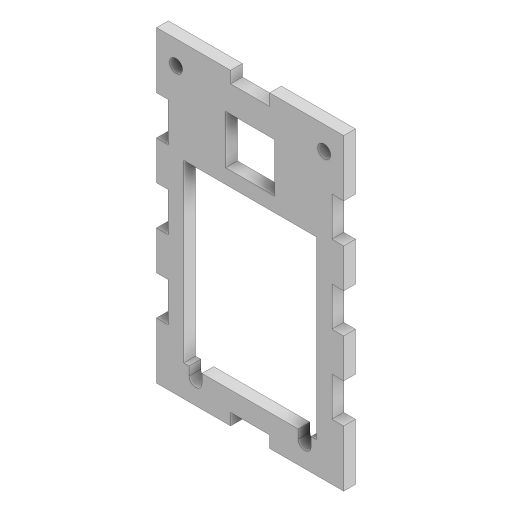
# Autodesk Inventor part: Top piece
Saved by Autodesk Inventor 2023.3 (Build 273359000, 359)
## iProperties
Created: 2024-09-20
Part Number: Top piece
Material: Generic
Document SubType Name: Modeling
Designer: David Zindović
Density: 1 g/cm^3
Appearance: Default
Author: David Zindović
Autodesk Inventor part; units mm, degrees
ref_plane "YZ Plane" through (0, 0, 0) normal (1, 0, 0) x (0, 1, 0)
ref_plane "XZ Plane" through (0, 0, 0) normal (0, 1, 0) x (-1, 0, 0)
ref_plane "XY Plane" through (0, 0, 0) normal (0, 0, 1) x (1, 0, 0)
sketch "Sketch1" plane through (0, 0, 0) normal (0, 0, 1) x (1, 0, 0)
  circle A0 centre (-14, -25.25) radius 1.65
  circle A1 centre (14, -25.25) radius 1.65
  circle A2 centre (-19, 42) radius 1.65
  circle A3 centre (19, 42) radius 1.65
  line L0 (-17, 22) -> (17, 22)
  line L1 (17, 22) -> (17, -22)
  line L2 (17, -22) -> (-17, -22)
  line L3 (-17, -22) -> (-17, 22)
  circle A4 centre (0, 32) radius 2.5
  line L4 (-24, 48) -> (24, 48)
  line L5 (24, 48) -> (24, -31)
  line L6 (24, -31) -> (-24, -31)
  line L7 (-24, -31) -> (-24, 48)
  line L8 (-17, -22) -> (17, -22)
  line L9 (17, -22) -> (17, -23)
  line L10 (17, -23) -> (-17, -23)
  line L11 (-17, -23) -> (-17, -22)
  line L12 (-15.65, -25.25) -> (-15.65, -23)
  line L13 (-12.35, -25.25) -> (-12.35, -23)
  line L14 (12.35, -25.25) -> (12.35, -23)
  line L15 (15.65, -25.25) -> (15.65, -23)
  line L16 (-24, 13.5) -> (-21, 13.5)
  line L17 (-21, 13.5) -> (-21, 3.5)
  line L18 (-21, 3.5) -> (-24, 3.5)
  line L19 (-24, 3.5) -> (-24, 13.5)
  line L20 (-5, -31) -> (5, -31)
  line L21 (5, -31) -> (5, -28)
  line L22 (5, -28) -> (-5, -28)
  line L23 (-5, -28) -> (-5, -31)
  line L24 (-5, 48) -> (5, 48)
  line L25 (5, 48) -> (5, 45)
  line L26 (5, 45) -> (-5, 45)
  line L27 (-5, 45) -> (-5, 48)
  line L28 (-21, 33.5) -> (-21, 23.5)
  line L29 (-21, 23.5) -> (-24, 23.5)
  line L30 (-24, 33.5) -> (-21, 33.5)
  line L31 (-21, -16.5) -> (-24, -16.5)
  line L32 (-21, -6.5) -> (-21, -16.5)
  line L33 (-24, -6.5) -> (-21, -6.5)
  line L34 (21, 13.5) -> (24, 13.5)
  line L35 (24, 13.5) -> (24, 3.5)
  line L36 (24, 3.5) -> (21, 3.5)
  line L37 (21, 3.5) -> (21, 13.5)
  line L38 (24, -16.5) -> (21, -16.5)
  line L39 (21, -16.5) -> (21, -6.5)
  line L40 (21, -6.5) -> (24, -6.5)
  line L41 (24, 23.5) -> (21, 23.5)
  line L42 (21, 23.5) -> (21, 33.5)
  line L43 (21, 33.5) -> (24, 33.5)
  line L44 (-6.25, 38.25) -> (6.25, 38.25)
  line L45 (6.25, 38.25) -> (6.25, 25.75)
  line L46 (6.25, 25.75) -> (-6.25, 25.75)
  line L47 (-6.25, 25.75) -> (-6.25, 38.25)
  point P0 (0, 0)
  point P1 (0, 22)
  point P2 (0, -22)
  point P3 (17, 0)
  point P4 (0, 48)
  point P5 (-24, 8.5)
  point P6 (0, -28)
  point P7 (0, -31)
  point P8 (0, -31)
  point P9 (0, 45)
  point P10 (24, 8.5)
  point P11 (24, 8.5)
  point P12 (0, 38.25)
  point P13 (6.25, 32)
  dimension "d0" = 3.3
  dimension "d1" = 3.3
  dimension "d2" = 28
  dimension "d3" = 14
  dimension "d4" = 3.3
  dimension "d5" = 3.3
  dimension "d6" = 38
  dimension "d7" = 19
  dimension "d8" = 34
  dimension "d9" = 44
  dimension "d10" = 3.25
  dimension "d11" = 20
  dimension "d12" = 5
  dimension "d13" = 10
  dimension "d14" = 9
  dimension "d15" = 26
  dimension "d16" = 7
  dimension "d17" = 1
  dimension "d18" = 3
  dimension "d19" = 10
  dimension "d20" = 10
  dimension "d21" = 3
  dimension "d22" = 10
  dimension "d23" = 3
  dimension "d26" = 20
  dimension "d33" = 20
  dimension "d38" = 3
  dimension "d39" = 10
  dimension "d42" = 20
  dimension "d49" = 20
  dimension "d56" = 12.5
  dimension "d57" = 12.5
  constraints: 96 end point, 16 parallel, 14 midpoint, 11 perpendicular, 8 horizontal, 8 vertical alignment, 6 point on line, 5 centre point, 5 vertical, 4 horizontal alignment, 4 point on circle, 4 tangent, 1 coincident, 1 collinear, 28 other
  measures "d0" diameter of A0
  measures "d1" diameter of A1
  measures "d2" distance of A1.centre A0.centre
  measures "d3" horizontal distance of point (0, 0) A0.centre
  measures "d4" diameter of A2
  measures "d5" diameter of A3
  measures "d6" distance of A3.centre A2.centre
  measures "d7" horizontal distance of point (0, 0) A2.centre
  measures "d8" distance of L1.end L2.end
  measures "d9" distance of L0.end L1.end
  measures "d10" distance from line of L2 A1.centre
  measures "d11" distance from line of L0 A2.centre
  measures "d12" diameter of A4
  measures "d13" distance from line of L0 A4.centre
  measures "d14" distance between parallel lines of L2 L6
  measures "d15" distance between parallel lines of L4 L0
  measures "d16" distance between parallel lines of L5 L1
  measures "d17" distance of L8.end L9.end
  measures "d18" distance of L17.end L18.end
  measures "d19" distance of L16.end L17.end
  measures "d20" distance of L21.end L22.end
  measures "d21" distance of L20.end L21.end
  measures "d22" distance of L25.end L26.end
  measures "d23" distance of L24.end L25.end
  measures "d26" distance of L16.end L28.start
  measures "d33" distance of L17.end L31.start
  measures "d38" distance of L35.end L36.end
  measures "d39" distance of L34.end L35.end
  measures "d42" distance of L36.end L38.end
  measures "d49" distance of L36.end L41.end
  measures "d56" distance of L45.end L46.end
  measures "d57" distance of L44.end L45.end
extrude "Extrusion1" add sketch "Sketch1" along normal mid plane 3 contours L4 L27 L26 L25 L5 L43 L42 L41 L34 L37 L36 L40 L39 L38 L6 L21 L22 L23 L7 L31 L32 L33 L18 L17 L16 L29 L28 L30
equation "\"d3\" = 0.5 * d2"
equation "\"d7\" = 0.5 * d6"
equation "\"d56\" = d57"
body "Solid1"
